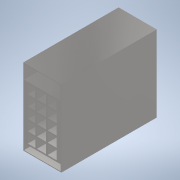
# Autodesk Inventor part: mainbox
Saved by Autodesk Inventor 2020.3 (Build 243373000, 373)
## iProperties
Created: 2021-08-07
Part Number: mainbox
Material: Stainless Steel
Document SubType Name: Modeling
Designer: 0x6f736f646f
Density: 8 g/cm^3
Appearance: Galvanized
Author: 0x6f736f646f
Autodesk Inventor part; units mm, degrees
ref_plane "YZ Plane" through (0, 0, 0) normal (1, 0, 0) x (0, 1, 0)
ref_plane "XZ Plane" through (0, 0, 0) normal (0, 1, 0) x (-1, 0, 0)
ref_plane "XY Plane" through (0, 0, 0) normal (0, 0, 1) x (1, 0, 0)
sketch "Sketch1" plane through (0, 0, 0) normal (0, 0, 1) x (1, 0, 0)
  line L0 (0, 0) -> (-200, 0)
  line L1 (-200, 400) -> (0, 400)
  line L2 (0, 400) -> (0, 0)
  line L3 (-136, 212) -> (-176, 212)
  line L4 (-136, 204) -> (-176, 204)
  line L5 (-80, 212) -> (-128, 212)
  line L6 (-80, 204) -> (-128, 204)
  line L7 (-196, 324) -> (-196, 396)
  line L8 (-180, 324) -> (-196, 324)
  line L9 (-180, 316) -> (-196, 316)
  line L10 (-136, 324) -> (-176, 324)
  line L11 (-136, 316) -> (-176, 316)
  line L12 (-4, 324) -> (-20, 324)
  line L13 (-4, 316) -> (-20, 316)
  line L14 (-24, 324) -> (-72, 324)
  line L15 (-80, 324) -> (-128, 324)
  line L16 (-24, 316) -> (-72, 316)
  line L17 (-80, 316) -> (-128, 316)
  line L18 (-20, 268) -> (-20, 316)
  line L19 (-24, 268) -> (-24, 316)
  line L20 (-24, 268) -> (-72, 268)
  line L21 (-72, 212) -> (-72, 260)
  line L22 (-72, 268) -> (-72, 316)
  line L23 (-24, 260) -> (-72, 260)
  line L24 (-80, 212) -> (-80, 260)
  line L25 (-80, 268) -> (-80, 316)
  line L26 (-80, 268) -> (-128, 268)
  line L27 (-136, 212) -> (-136, 260)
  line L28 (-136, 268) -> (-136, 316)
  line L29 (-80, 260) -> (-128, 260)
  line L30 (-128, 212) -> (-128, 260)
  line L31 (-128, 268) -> (-128, 316)
  line L32 (-136, 268) -> (-176, 268)
  line L33 (-136, 260) -> (-176, 260)
  line L34 (-196, 212) -> (-196, 260)
  line L35 (-196, 268) -> (-196, 316)
  line L36 (-180, 212) -> (-180, 260)
  line L37 (-180, 268) -> (-180, 316)
  line L38 (-176, 212) -> (-176, 260)
  line L39 (-176, 268) -> (-176, 316)
  line L40 (-200, 0) -> (-200, 152)
  line L41 (-200, 156) -> (-200, 400)
  line L42 (-180, 44) -> (-196, 44)
  line L43 (-136, 44) -> (-176, 44)
  line L44 (-80, 44) -> (-128, 44)
  line L45 (-4, 4) -> (-20, 4)
  line L46 (-180, 4) -> (-196, 4)
  line L47 (-80, 44) -> (-80, 92)
  line L48 (-72, 44) -> (-72, 92)
  line L49 (-128, 44) -> (-128, 92)
  line L50 (-80, 100) -> (-128, 100)
  line L51 (-136, 44) -> (-136, 92)
  line L52 (-80, 92) -> (-128, 92)
  line L53 (-24, 100) -> (-72, 100)
  line L54 (-24, 92) -> (-72, 92)
  line L55 (-24, 100) -> (-24, 148)
  line L56 (-20, 100) -> (-20, 148)
  line L57 (-4, 148) -> (-4, 100)
  line L58 (-72, 100) -> (-72, 148)
  line L59 (-72, 156) -> (-72, 204)
  line L60 (-80, 100) -> (-80, 148)
  line L61 (-80, 156) -> (-80, 204)
  line L62 (-24, 156) -> (-72, 156)
  line L63 (-24, 148) -> (-72, 148)
  line L64 (-128, 100) -> (-128, 148)
  line L65 (-128, 156) -> (-128, 204)
  line L66 (-80, 156) -> (-128, 156)
  line L67 (-136, 100) -> (-136, 148)
  line L68 (-136, 156) -> (-136, 204)
  line L69 (-80, 148) -> (-128, 148)
  line L70 (-136, 156) -> (-176, 156)
  line L71 (-136, 148) -> (-176, 148)
  line L72 (-180, 156) -> (-180, 204)
  line L73 (-176, 156) -> (-176, 204)
  line L74 (-196, 156) -> (-196, 204)
  line L75 (-20, 396) -> (-4, 396)
  line L76 (-72, 396) -> (-24, 396)
  line L77 (-128, 396) -> (-80, 396)
  line L78 (-196, 396) -> (-180, 396)
  line L79 (-176, 396) -> (-136, 396)
  line L80 (-136, 100) -> (-176, 100)
  line L81 (-136, 92) -> (-176, 92)
  line L82 (-180, 44) -> (-180, 92)
  line L83 (-180, 100) -> (-180, 148)
  line L84 (-176, 44) -> (-176, 92)
  line L85 (-176, 100) -> (-176, 148)
  line L86 (-196, 44) -> (-196, 92)
  line L87 (-196, 100) -> (-196, 148)
  line L88 (-4, 44) -> (-20, 44)
  line L89 (-24, 44) -> (-72, 44)
  line L90 (-24, 44) -> (-24, 92)
  line L91 (-20, 44) -> (-20, 92)
  line L92 (-4, 92) -> (-4, 44)
  line L93 (-4, 396) -> (-4, 324)
  line L94 (-4, 316) -> (-4, 268)
  line L95 (-180, 396) -> (-176, 396)
  line L96 (-136, 396) -> (-128, 396)
  line L97 (-80, 396) -> (-72, 396)
  line L98 (-24, 396) -> (-20, 396)
  line L99 (-20, 324) -> (-24, 324)
  line L100 (-72, 324) -> (-80, 324)
  line L101 (-128, 324) -> (-136, 324)
  line L102 (-176, 324) -> (-180, 324)
  line L103 (-200, 152) -> (-200, 156)
  line L104 (-24, 212) -> (-72, 212)
  line L105 (-24, 156) -> (-24, 204)
  line L106 (-24, 212) -> (-24, 260)
  line L107 (-24, 204) -> (-72, 204)
  line L108 (-20, 156) -> (-20, 204)
  line L109 (-20, 212) -> (-20, 260)
  line L110 (-4, 260) -> (-4, 212)
  line L111 (-4, 204) -> (-4, 156)
  line L112 (-4, 4) -> (-196, 4)
  line L113 (-196, 4) -> (-196, 36)
  line L114 (-196, 36) -> (-4, 36)
  line L115 (-4, 36) -> (-4, 4)
  line L116 (-180, 44) -> (-196, 44)
  line L117 (-196, 44) -> (-196, 316)
  line L118 (-196, 316) -> (-180, 316)
  line L119 (-180, 316) -> (-180, 44)
  line L120 (-20, 316) -> (-4, 316)
  line L121 (-4, 316) -> (-4, 44)
  line L122 (-4, 44) -> (-20, 44)
  line L123 (-20, 44) -> (-20, 316)
  point P0 (-20, 4)
  point P1 (-180, 4)
  dimension "d0" = 200
  dimension "d1" = 400
  dimension "d32" = 4
  dimension "d33" = 16
  dimension "d34" = 4
  dimension "d35" = 40
  dimension "d36" = 4
  dimension "d37" = 20
  dimension "d38" = 4
  dimension "d39" = 48
  dimension "d40" = 8
  dimension "d41" = 48
  dimension "d42" = 48
  dimension "d43" = 4
  dimension "d44" = 32
  dimension "d45" = 192
  dimension "d46" = 4
  dimension "d47" = 4
  constraints: 248 end point, 105 parallel, 35 equal length, 23 perpendicular, 7 collinear, 5 horizontal
  measures "d0" distance of L1.start L1.end
  measures "d1" distance of L0.end L1.start
  measures "d32" distance between parallel lines of L35 L41
  measures "d33" distance between parallel lines of L37 L35
  measures "d34" distance between parallel lines of L39 L37
  measures "d35" distance between parallel lines of L39 L28
  measures "d36" distance between parallel lines of L2 L94
  measures "d37" distance between parallel lines of L2 L18
  measures "d38" distance between parallel lines of L18 L19
  measures "d39" distance between parallel lines of L19 L22
  measures "d40" distance between parallel lines of L22 L25
  measures "d41" distance between parallel lines of L25 L31
  measures "d42" distance between parallel lines of L26 L17
  measures "d43" distance between parallel lines of L110 L2
  measures "d44" distance of L112.end L113.end
  measures "d45" distance between parallel lines of L115 L113
  measures "d46" distance between parallel lines of L2 L115
  measures "d47" distance between parallel lines of L0 L112
extrude "Extrusion1" add sketch "Sketch1" along normal blind 250 contours L0 L40 L103 L41 L1 L2 | L37 L119 L36 L72 L83 L82 L42 L86 L117 L87 L74 L34 L35 L9 | L94 L121 L110 L111 L57 L92 L88 L91 L123 L56 L108 L109 L18 L13
extrude "Extrusion2" add sketch "Sketch1" along normal blind 50 contours L0 L40 L103 L41 L1 L2 | L3 L38 L33 L27 | L68 L70 L73 L4 | L5 L30 L29 L24 | L61 L66 L65 L6 | L7 L78 L95 L79 L96 L77 L97 L76 L98 L75 L93 L12 L99 L14 L100 L15 L101 L10 L102 L8 | L37 L119 L36 L72 L83 L82 L42 L86 L117 L87 L74 L34 L35 L9 | L28 L32 L39 L11 | L94 L121 L110 L111 L57 L92 L88 L91 L123 L56 L108 L109 L18 L13 | L19 L20 L22 L16 | L25 L26 L31 L17 | L21 L23 L106 L104 | L43 L84 L81 L51 | L44 L49 L52 L47 | L45 L112 L46 L113 L114 L115 | L48 L54 L90 L89 | L50 L64 L69 L60 | L53 L58 L63 L55 | L59 L107 L105 L62 | L80 L85 L71 L67
body "Solid1"
